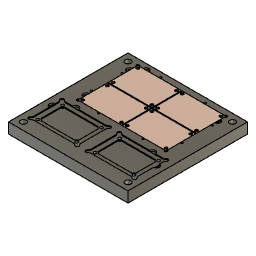
4x6 PCB jig (Autodesk Fusion 360 design; units mm, degrees)
Autodesk Fusion 360 part; units mm, degrees
sketch "Sketch1" plane through (0, 0, 0) normal (0, 0, 1) x (1, 0, 0) in component "holder"
  line L0 (0, 0) -> (203.2, 0)
  line L1 (203.2, 0) -> (203.2, 203.2)
  line L2 (203.2, 203.2) -> (0, 203.2)
  line L3 (0, 203.2) -> (0, 0)
  circle A0 centre (12.7, 12.7) radius 3
  circle A1 centre (190.5, 12.7) radius 3
  circle A2 centre (12.7, 190.5) radius 3
  circle A3 centre (190.5, 190.5) radius 3
  circle A4 centre (12.7, 12.7) radius 5
  circle A5 centre (190.5, 12.7) radius 5
  circle A6 centre (12.7, 190.5) radius 5
  circle A7 centre (190.5, 190.5) radius 5
  dimension "d1" = 203.2
  dimension "d2" = 203.2
  dimension "d3" = 6
  dimension "d4" = 12.7
  dimension "d5" = 12.7
  dimension "d8" = 177.8
  dimension "d9" = 177.8
  dimension "d12" = 10
  dimension "d15" = 177.8
  dimension "d16" = 177.8
  constraint horizontal L0
  constraint vertical L1
  constraint horizontal L2
  constraint vertical L3
  constraint coincident L0.start L3.end
  constraint concentric A0 A4
  measures "d1" distance of L0.start L0.end
  measures "d2" distance of L0.start L2.end
  measures "d3" diameter of A0
  measures "d4" distance of L3 A0.centre
  measures "d5" distance of L0 A0.centre
  measures "d12" diameter of A4
extrude "Extrude1" add sketch "Sketch1" along normal blind 17.9 contours L0 L1 L2 L3 | A4 | A5 | A6 | A7 makes body 1 in component "holder"
extrude "Extrude2" cut sketch "Sketch1" against normal blind 6.5 from surface at 17.9 contours A4 | A5 | A6 | A7 bodies 1 in component "holder"
sketch "Sketch2" plane through (0, 0, 17.9) normal (0, 0, 1) x (-1, 0, 0) in component "holder"
  circle A0 centre (-190.5, -12.7) radius 5
  circle A1 centre (-190.5, -190.5) radius 5
  circle A2 centre (-12.7, -12.7) radius 5
  circle A3 centre (-12.7, -190.5) radius 5
  line L0 (0, -203.2) -> (0, 0)
  line L1 (0, 0) -> (-203.2, 0)
  line L2 (-203.2, 0) -> (-203.2, -203.2)
  line L3 (-203.2, -203.2) -> (0, -203.2)
  line L4 (-26.7, -193.2) -> (-176.5, -193.2)
  line L5 (-176.5, -193.2) -> (-176.5, -91.3)
  line L6 (-176.5, -91.3) -> (-26.7, -91.3)
  line L7 (-26.7, -91.3) -> (-26.7, -193.2)
  line L8 (0, -203.2) -> (0, 0)
  line L9 (0, 0) -> (-203.2, 0)
  line L10 (-203.2, -203.2) -> (0, -203.2)
  line L11 (-13, -78) -> (-93, -78) construction
  line L12 (-93, -78) -> (-93, -24) construction
  line L13 (-93, -24) -> (-13, -24) construction
  line L14 (-13, -24) -> (-13, -78) construction
  line L15 (-101.6, -203.2) -> (-101.6, 0)
  line L16 (-53, -78) -> (-53, -24) construction
  line L17 (-13, -51) -> (-93, -51) construction
  line L18 (-13, -51) -> (-13.0014, -30.2465)
  line L19 (-53, -24) -> (-19.2578, -24.0135)
  arc A4 (-11.1255, -26.3423) -> (-15.3459, -22.1301) centre (-13, -24) ccw
  arc A5 (-11.1255, -26.3423) -> (-13.0014, -30.2465) centre (-8.0014, -30.2461) ccw
  arc A6 (-19.2578, -24.0135) -> (-15.3459, -22.1301) centre (-19.2558, -19.0135) ccw
  line L20 (-93, -51) -> (-92.9986, -30.2465)
  arc A7 (-92.9986, -30.2465) -> (-94.8745, -26.3423) centre (-97.9986, -30.2461) ccw
  arc A8 (-90.6541, -22.1301) -> (-94.8745, -26.3423) centre (-93, -24) ccw
  arc A9 (-90.6541, -22.1301) -> (-86.7422, -24.0135) centre (-86.7442, -19.0135) ccw
  line L21 (-53, -24) -> (-86.7422, -24.0135)
  line L22 (-53, -78) -> (-86.7422, -77.9865)
  arc A10 (-86.7422, -77.9865) -> (-90.6541, -79.8699) centre (-86.7442, -82.9865) ccw
  arc A11 (-94.8745, -75.6577) -> (-90.6541, -79.8699) centre (-93, -78) ccw
  arc A12 (-94.8745, -75.6577) -> (-92.9986, -71.7535) centre (-97.9986, -71.7539) ccw
  line L23 (-93, -51) -> (-92.9986, -71.7535)
  line L24 (-13, -51) -> (-13.0014, -71.7535)
  arc A13 (-13.0014, -71.7535) -> (-11.1255, -75.6577) centre (-8.0014, -71.7539) ccw
  arc A14 (-15.3459, -79.8699) -> (-19.2578, -77.9865) centre (-19.2558, -82.9865) ccw
  line L25 (-53, -78) -> (-19.2578, -77.9865)
  arc A15 (-15.3459, -79.8699) -> (-11.1255, -75.6577) centre (-13, -78) ccw
  line L26 (-26.7, -142.25) -> (-176.5, -142.25) construction
  arc A16 (-28.7, -193.2) -> (-26.7, -191.2) centre (-26.7, -193.2) ccw
  arc A17 (-176.5, -191.2) -> (-174.5, -193.2) centre (-176.5, -193.2) ccw
  arc A18 (-174.5, -91.3) -> (-176.5, -93.3) centre (-176.5, -91.3) ccw
  arc A19 (-26.7, -93.3) -> (-28.7, -91.3) centre (-26.7, -91.3) ccw
  circle A20 centre (-24.94, -168.1) radius 1.675
  line L27 (-26.7, -168.1) -> (-176.5, -168.1) construction
  line L28 (-63.775, -193.2) -> (-63.775, -91.3) construction
  line L29 (-26.7, -168.1) -> (-16.7, -168.1) construction
  line L30 (-63.775, -193.2) -> (-63.775, -203.2) construction
  circle A21 centre (-63.775, -194.96) radius 1.675
  circle A22 centre (-63.775, -89.54) radius 1.675
  circle A23 centre (-24.94, -116.4) radius 1.675
  circle A24 centre (-139.425, -194.96) radius 1.675
  circle A25 centre (-178.26, -168.1) radius 1.675
  circle A26 centre (-178.26, -116.4) radius 1.675
  circle A27 centre (-139.425, -89.54) radius 1.675
  circle A28 centre (-30.775, -189.1) radius 2.425
  circle A29 centre (-96.775, -189.1) radius 2.425
  circle A30 centre (-30.775, -147.1) radius 2.425
  circle A31 centre (-96.775, -147.1) radius 2.425
  line L31 (-100.85, -193.2) -> (-100.85, -91.3) construction
  arc A32 (-100.85, -91.3) -> (-102.35, -91.3) centre (-101.6, -91.3) ccw construction
  line L32 (-102.35, -91.3) -> (-102.35, -193.2) construction
  arc A33 (-102.35, -193.2) -> (-100.85, -193.2) centre (-101.6, -193.2) ccw construction
  line L33 (-101.6, -193.2) -> (-101.6, -91.3) construction
  line L34 (-26.7, -141.5) -> (-176.5, -141.5) construction
  arc A34 (-176.5, -141.5) -> (-176.5, -143) centre (-176.5, -142.25) ccw construction
  line L35 (-176.5, -143) -> (-26.7, -143) construction
  arc A35 (-26.7, -143) -> (-26.7, -141.5) centre (-26.7, -142.25) ccw construction
  line L36 (-26.7, -142.25) -> (-176.5, -142.25)
  circle A36 centre (-172.425, -189.1) radius 2.425
  circle A37 centre (-106.425, -189.1) radius 2.425
  circle A38 centre (-106.425, -147.1) radius 2.425
  circle A39 centre (-172.425, -147.1) radius 2.425
  circle A40 centre (-30.775, -95.4) radius 2.425
  circle A41 centre (-96.775, -95.4) radius 2.425
  circle A42 centre (-106.425, -95.4) radius 2.425
  circle A43 centre (-172.425, -95.4) radius 2.425
  circle A44 centre (-172.425, -137.4) radius 2.425
  circle A45 centre (-106.425, -137.4) radius 2.425
  circle A46 centre (-96.775, -137.4) radius 2.425
  circle A47 centre (-30.775, -137.4) radius 2.425
  circle A48 centre (-20, -72) radius 2.425
  circle A49 centre (-86, -72) radius 2.425
  circle A50 centre (-20, -30) radius 2.425
  circle A51 centre (-86, -30) radius 2.425
  line L37 (-150.2, -78) -> (-183.9422, -77.9865)
  arc A52 (-183.9422, -77.9865) -> (-187.8541, -79.8699) centre (-183.9442, -82.9865) ccw
  arc A53 (-192.0745, -75.6577) -> (-190.1986, -71.7535) centre (-195.1986, -71.7539) ccw
  line L38 (-190.2, -51) -> (-190.1986, -71.7535)
  arc A54 (-192.0745, -75.6577) -> (-187.8541, -79.8699) centre (-190.2, -78) ccw
  line L39 (-110.2, -51) -> (-110.2014, -71.7535)
  arc A55 (-110.2014, -71.7535) -> (-108.3255, -75.6577) centre (-105.2014, -71.7539) ccw
  arc A56 (-112.5459, -79.8699) -> (-116.4578, -77.9865) centre (-116.4558, -82.9865) ccw
  line L40 (-150.2, -78) -> (-116.4578, -77.9865)
  arc A57 (-112.5459, -79.8699) -> (-108.3255, -75.6577) centre (-110.2, -78) ccw
  line L41 (-150.2, -24) -> (-116.4578, -24.0135)
  arc A58 (-116.4578, -24.0135) -> (-112.5459, -22.1301) centre (-116.4558, -19.0135) ccw
  arc A59 (-108.3255, -26.3423) -> (-110.2014, -30.2465) centre (-105.2014, -30.2461) ccw
  line L42 (-110.2, -51) -> (-110.2014, -30.2465)
  arc A60 (-108.3255, -26.3423) -> (-112.5459, -22.1301) centre (-110.2, -24) ccw
  line L43 (-190.2, -51) -> (-190.1986, -30.2465)
  arc A61 (-190.1986, -30.2465) -> (-192.0745, -26.3423) centre (-195.1986, -30.2461) ccw
  arc A62 (-187.8541, -22.1301) -> (-183.9422, -24.0135) centre (-183.9442, -19.0135) ccw
  line L44 (-150.2, -24) -> (-183.9422, -24.0135)
  arc A63 (-187.8541, -22.1301) -> (-192.0745, -26.3423) centre (-190.2, -24) ccw
  circle A64 centre (-183.2, -30) radius 2.425
  circle A65 centre (-183.2, -72) radius 2.425
  circle A66 centre (-117.2, -72) radius 2.425
  circle A67 centre (-117.2, -30) radius 2.425
  circle A68 centre (-20, -72) radius 3.545
  circle A69 centre (-86, -72) radius 3.545
  circle A70 centre (-20, -30) radius 3.545
  circle A71 centre (-86, -30) radius 3.545
  circle A72 centre (-183.2, -72) radius 3.545
  circle A73 centre (-117.2, -72) radius 3.545
  circle A74 centre (-117.2, -30) radius 3.545
  circle A75 centre (-183.2, -30) radius 3.545
  line L45 (-27.6816, -194.9425) -> (-30.775, -193.2)
  line L46 (-24.9541, -192.2244) -> (-26.7, -189.1)
  line L47 (-175.5184, -194.9425) -> (-172.425, -193.2)
  line L48 (-178.2459, -192.2244) -> (-176.5, -189.1)
  line L49 (-24.9541, -92.2756) -> (-26.7, -95.4)
  line L50 (-27.6816, -89.5575) -> (-30.775, -91.3)
  line L51 (-175.5184, -89.5575) -> (-172.425, -91.3)
  line L52 (-178.2459, -92.2756) -> (-176.5, -95.4)
  dimension "d20" = 149.8
  dimension "d21" = 101.9
  dimension "d24" = 10
  dimension "d25" = 80
  dimension "d26" = 54
  dimension "d30" = 6
  dimension "d31" = 5
  dimension "d32" = 4
  dimension "d33" = 3.35
  dimension "d34" = 1.76
  dimension "d37" = 1.76
  dimension "d38" = 4.85
  dimension "d39" = 66
  dimension "d40" = 42
  dimension "d41" = 1.5
  dimension "d42" = 1.5
  dimension "d43" = 66
  dimension "d44" = 42
  dimension "d45" = 20
  dimension "d46" = 30
  dimension "d47" = 7.09
  constraint horizontal L4
  constraint vertical L5
  constraint horizontal L6
  constraint vertical L7
  constraint horizontal L11
  constraint vertical L12
  constraint horizontal L13
  constraint vertical L14
  constraint midpoint L3 L15.start
  constraint midpoint L1 L15.end
  constraint midpoint L11 L16.start
  constraint midpoint L13 L16.end
  constraint midpoint L14 L17.start
  constraint midpoint L12 L17.end
  constraint coincident L13.end L14.start
  constraint tangent L18 A5
  constraint tangent A4 A5
  constraint tangent L19 A6
  constraint tangent A4 A6
  constraint equal A5 A6
  constraint symmetric L19.start L16 L21.start
  constraint symmetric L16 L17.start L17.end
  constraint symmetric L16 A4 A8
  constraint symmetric L16 L18.end L20.end
  constraint symmetric L16 A4.start A7.end
  constraint symmetric L16 A5 A7
  constraint symmetric L16 L19.end A9.end
  constraint symmetric L16 A4.end A8.start
  constraint symmetric L16 A6 A9
  constraint symmetric L16.end L17 L16.start
  constraint symmetric L18.start L17 L24.start
  constraint symmetric L17 A4 A15
  constraint symmetric L17 L18.end L24.end
  constraint symmetric L17 A4.start A13.end
  constraint symmetric L17 A5 A13
  constraint symmetric L17 L19.end A14.end
  constraint symmetric L17 A4.end A14.start
  constraint symmetric L17 A6 A14
  constraint symmetric L17 L20.start L23.start
  constraint symmetric L17 L20.end A12.end
  constraint symmetric L17 A7.end A11.start
  constraint symmetric L17 A7 A12
  constraint symmetric L17 A8.start A10.end
  constraint symmetric L17 A8 A11
  constraint symmetric L17 A9.end L22.end
  constraint symmetric L17 A9 A10
  constraint symmetric L17 L16.end L16.start
  constraint symmetric L5 L7 L15
  constraint coincident L4.start L7.end
  constraint symmetric L15 A16 A17
  constraint midpoint L7 L26.start
  constraint midpoint L5 L26.end
  constraint symmetric L26 A16 A19
  constraint symmetric L26 A17 A18
  constraint coincident L7 A16.end
  constraint coincident L4 A16.start
  constraint coincident L4 A17.end
  constraint coincident L5 A17.start
  constraint coincident L5 A18.end
  constraint coincident L6 A18.start
  constraint coincident L6 A19.end
  constraint coincident L7 A19.start
  constraint coincident L7 L27.start
  constraint coincident L5 L27.end
  constraint perpendicular L5 L27
  constraint coincident L4 L28.start
  constraint coincident L6 L28.end
  constraint perpendicular L7 L29
  constraint perpendicular L4 L30
  constraint coincident A20.centre L29
  constraint equal A20 A21
  constraint coincident L30 A21.centre
  constraint symmetric L26 A20 A23
  constraint symmetric L26 A21 A22
  constraint symmetric L15 A20 A25
  constraint symmetric L15 A21 A24
  constraint symmetric L15 A22 A27
  constraint symmetric L15 A23 A26
  constraint symmetric L27 A28 A30
  constraint tangent L31 A32
  constraint tangent A32 L32
  constraint parallel L31 L32
  constraint tangent L32 A33
  constraint tangent L31 A33
  constraint midpoint L6 A32.centre
  constraint perpendicular L6 L33
  constraint midpoint L4 A33.centre
  constraint tangent L34 A34
  constraint tangent A34 L35
  constraint parallel L34 L35
  constraint tangent L35 A35
  constraint tangent L34 A35
  constraint coincident L26.end A34.centre
  constraint perpendicular L5 L36
  constraint coincident L26.start A35.centre
  constraint symmetric L4 L27 L35
  constraint symmetric L28 A28.centre A29.centre
  constraint equal A28 A29
  constraint equal A28 A31
  constraint vertical A29.centre A31.centre
  constraint horizontal A30.centre A31.centre
  constraint symmetric L15 A28 A36
  constraint symmetric L15 A29 A37
  constraint symmetric L15 A30 A39
  constraint symmetric L15 A31 A38
  constraint symmetric A28 L36 A40
  constraint symmetric A29 L36 A41
  constraint symmetric A30 L36 A47
  constraint symmetric A31 L36 A46
  constraint symmetric L36 A36 A43
  constraint symmetric L36 A37 A42
  constraint symmetric L36 A38 A45
  constraint symmetric L36 A39 A44
  constraint equal A28 A48
  constraint symmetric L16 A48 A49
  constraint symmetric L17 A48 A50
  constraint symmetric L17 A49 A51
  constraint symmetric L15 L16.end L41.start
  constraint symmetric L15 L17.start L38.start
  constraint symmetric L15 A4 A63
  constraint symmetric L15 L18.end L43.end
  constraint symmetric L15 A4.start A61.end
  constraint symmetric L15 A5 A61
  constraint symmetric L15 L19.end A62.end
  constraint symmetric L15 A4.end A62.start
  constraint symmetric L15 A6 A62
  constraint symmetric L15 L17.end L39.start
  constraint symmetric L15 L20.end A59.end
  constraint symmetric L15 A7.end A59.start
  constraint symmetric L15 A7 A59
  constraint symmetric L15 A8.start A58.end
  constraint symmetric L15 A8 A60
  constraint symmetric L15 A9.end L41.end
  constraint symmetric L15 A9 A58
  constraint symmetric L15 L16.start L37.start
  constraint symmetric L15 L22.end A56.end
  constraint symmetric L15 A10.end A56.start
  constraint symmetric L15 A10 A56
  constraint symmetric L15 A11.start A55.end
  constraint symmetric L15 A11 A57
  constraint symmetric L15 A12.end L39.end
  constraint symmetric L15 A12 A55
  constraint symmetric L15 L24.end A53.end
  constraint symmetric L15 A13.end A53.start
  constraint symmetric L15 A13 A53
  constraint symmetric L15 A14.end L37.end
  constraint symmetric L15 A14.start A52.end
  constraint symmetric L15 A14 A52
  constraint symmetric L15 A15 A54
  constraint symmetric L15 A48 A65
  constraint symmetric L15 A49 A66
  constraint symmetric L15 A50 A64
  constraint symmetric L15 A51 A67
  constraint concentric A48 A68
  constraint symmetric L16 A68 A69
  constraint symmetric L17 A68 A70
  constraint symmetric L17 A69 A71
  constraint symmetric L15 A68 A72
  constraint symmetric L15 A69 A73
  constraint symmetric L15 A70 A75
  constraint symmetric L15 A71 A74
  constraint coincident A16 L45.start
  constraint coincident L4 L45.end
  constraint tangent A16 L45
  constraint vertical A28.centre L45.end
  constraint coincident A16 L46.start
  constraint tangent A16 L46
  constraint horizontal A28.centre L46.end
  constraint coincident L7 L46.end
  constraint symmetric L15 L45.start L47.start
  constraint symmetric L15 L45.end L47.end
  constraint symmetric L15 L46.start L48.start
  constraint symmetric L15 L46.end L48.end
  constraint symmetric L26 L45.start L50.start
  constraint symmetric L26 L45.end L50.end
  constraint symmetric L26 L46.start L49.start
  constraint symmetric L26 L46.end L49.end
  constraint symmetric L26 L47.start L51.start
  constraint symmetric L26 L47.end L51.end
  constraint symmetric L26 L48.start L52.start
  constraint symmetric L26 L48.end L52.end
  measures "d20" distance of L4.start L4.end
  measures "d21" distance of L4.start L6.end
  measures "d24" distance of L4 L10
  measures "d25" distance of L11.start L11.end
  measures "d26" distance of L11.start L13.end
  measures "d30" diameter of A4
  measures "d31" radius of A5
  measures "d32" diameter of A16
  measures "d33" diameter of A20
  measures "d34" distance of L7 A20.centre
  measures "d37" vertical distance of L28.start A21.centre
  measures "d38" diameter of A28
  measures "d39" distance of A28.centre A29.centre
  measures "d40" distance of A28.centre A30.centre
  measures "d41" diameter of A32
  measures "d42" diameter of A34
  measures "d43" distance of A48.centre A49.centre
  measures "d44" distance of A48.centre A50.centre
  measures "d45" distance of L8 A50.centre
  measures "d46" distance of L9 A50.centre
  measures "d47" diameter of A68
extrude "Extrude3" cut sketch "Sketch2" against normal blind 1.5 contours L4 L7 L15 L36 | L4 L5 L15 L36 | L5 L6 L15 L36 | L6 L7 L15 L36 | L4 A16 L45 | L4 A17 L47 | L6 A18 L51 | L6 A19 L50 | L4 L7 A16 | L4 L5 A17 | L5 L6 A18 | L6 L7 A19 | L7 A16 L46 | L5 A17 L48 | L7 A19 L49 | L5 A18 L52 | L18 L19 A4 A5 A6 L20 A7 A8 A9 L21 L22 A10 A11 A12 L23 L24 A13 A14 L25 A15 | A28 | A29 | A30 | A31 | A36 | A37 | A38 | A39 | A40 | A41 | A42 | A43 | A44 | A45 | A46 | A47 | A48 | A49 | A50 | A51 | L37 A52 A53 L38 A54 L39 A55 A56 L40 A57 L41 A58 A59 L42 A60 L43 A61 A62 L44 A63 | A64 | A65 | A66 | A67 | A68 | A69 | A70 | A71 | A72 | A73 | A74 | A75 bodies 1 in component "holder"
sketch "Sketch1 (2)" plane through (0, 0, 0) normal (1, 0, 0) x (0, 1, 0)
extrude "Extrude4" cut sketch "Sketch2" against normal blind 12 contours A20 | A21 | A22 | A23 | A24 | A25 | A26 | A27 bodies 1 in component "holder"
extrude "Extrude5" cut sketch "Sketch2" against normal blind 4 contours A28 | A29 | A30 | A31 | A36 | A37 | A38 | A39 | A40 | A41 | A42 | A43 | A44 | A45 | A46 | A47 bodies 1 in component "holder"
extrude "Extrude6" cut sketch "Sketch2" against normal up to surface (17.9 mm away) contours A48 | A49 | A50 | A51 | A64 | A65 | A66 | A67 bodies 1 in component "holder"
extrude "Extrude7" cut sketch "Sketch2" along normal blind 9.5 from surface at -17.9 contours A68 | A69 | A70 | A71 | A72 | A73 | A74 | A75 bodies 1 in component "holder"
sketch "Sketch2 (2)" plane through (0, 0, 0) normal (0, 0, -1) x (1, 0, 0)
  circle A0 centre (117.2, -30) radius 3.545
  circle A1 centre (86, -72) radius 3.545
  circle A2 centre (86, -30) radius 3.545
  circle A3 centre (183.2, -30) radius 3.545
  circle A4 centre (117.2, -72) radius 3.545
  circle A5 centre (20, -72) radius 3.545
  circle A6 centre (20, -30) radius 3.545
  circle A7 centre (183.2, -72) radius 3.545
  circle A8 centre (12.7, -190.5) radius 3
  circle A9 centre (190.5, -190.5) radius 3
  circle A10 centre (190.5, -12.7) radius 3
  circle A11 centre (12.7, -12.7) radius 3
  line L0 (0, 0) -> (0, -203.2)
  line L1 (0, -203.2) -> (203.2, -203.2)
  line L2 (203.2, -203.2) -> (203.2, 0)
  line L3 (203.2, 0) -> (0, 0)
sketch "Sketch3" plane through (0, 0, 17.9) normal (0, 0, 1) x (-1, 0, 0)
  line L0 (-26.7, -91.3) -> (-26.7, -193.2)
  line L1 (-13, -51) -> (-13.0014, -71.7535)
  line L2 (-53, -78) -> (-19.2578, -77.9865)
  line L3 (-190.2, -51) -> (-190.1986, -71.7535)
  line L4 (-150.2, -78) -> (-183.9422, -77.9865)
  line L5 (-176.5, -91.3) -> (-26.7, -91.3)
  line L6 (-176.5, -193.2) -> (-176.5, -91.3)
  line L7 (-53, -24) -> (-19.2578, -24.0135)
  line L8 (-13, -24) -> (-13, -78)
  line L9 (-150.2, -24) -> (-183.9422, -24.0135)
  line L10 (-190.2, -51) -> (-190.1986, -30.2465)
  circle A0 centre (-26.7, -179.2) radius 5
  line L11 (-26.7, -193.2) -> (-176.5, -193.2)
  circle A1 centre (-40.7, -193.2) radius 5
  circle A2 centre (-26.7, -105.3) radius 5
  circle A3 centre (-13.0007, -61.3768) radius 5
  circle A4 centre (-36.1289, -77.9932) radius 5
  circle A5 centre (-167.0711, -77.9932) radius 5
  circle A6 centre (-190.1993, -61.3768) radius 5
  circle A7 centre (-176.5, -179.2) radius 5
  dimension "d59" = 10
  dimension "d60" = 14
  dimension "d61" = 10
  dimension "d62" = 14
  dimension "d63" = 10
  dimension "d64" = 14
  dimension "d65" = 10
  dimension "d66" = 10
  dimension "d67" = 10
  dimension "d68" = 10
  dimension "d69" = 10
  constraint coincident L0 A0.centre
  constraint coincident L11 A1.centre
  constraint coincident L0 A2.centre
  constraint midpoint L1 A3.centre
  constraint midpoint L2 A4.centre
  constraint midpoint L4 A5.centre
  constraint midpoint L3 A6.centre
  constraint coincident L6 A7.centre
  constraint horizontal A0.centre A7.centre
  measures "d59" diameter of A0
  measures "d60" distance of A0.centre L11
  measures "d61" diameter of A1
  measures "d62" distance of L0 A1.centre
  measures "d63" diameter of A2
  measures "d64" distance of L5 A2.centre
  measures "d65" diameter of A3
  measures "d66" diameter of A4
  measures "d67" diameter of A5
  measures "d68" diameter of A6
  measures "d69" diameter of A7
extrude "Extrude8" cut sketch "Sketch3" against normal blind 2.5 contours L0 A2 | L6 A7 | L0 A0 | L11 A1 | L8 A3 | L2 A4 | L3 A6 | L4 A5 picked at (-24.7337, -106.442) picked at (-177.4715, -180.683) picked at (-23.6872, -180.4506) picked at (-42.1373, -195.7637) picked at (-34.8883, -79.3751) picked at (-191.3865, -62.7725) picked at (-165.7533, -81.1536) bodies 1 in component "holder"
sketch "Sketch3 (2)" plane through (0, 0, 16.4) normal (0, 0, 1) x (-1, 0, 0) in component "holder"
  circle A0 centre (-30.775, -95.4) radius 2.425
  circle A1 centre (-106.425, -189.1) radius 2.425
  circle A2 centre (-172.425, -189.1) radius 2.425
  circle A3 centre (-96.775, -189.1) radius 2.425
  circle A4 centre (-30.775, -147.1) radius 2.425
  circle A5 centre (-172.425, -137.4) radius 2.425
  circle A6 centre (-96.775, -147.1) radius 2.425
  circle A7 centre (-96.775, -95.4) radius 2.425
  circle A8 centre (-172.425, -95.4) radius 2.425
  circle A9 centre (-30.775, -189.1) radius 2.425
  circle A10 centre (-106.425, -147.1) radius 2.425
  circle A11 centre (-30.775, -137.4) radius 2.425
  circle A12 centre (-172.425, -147.1) radius 2.425
  circle A13 centre (-106.425, -137.4) radius 2.425
  circle A14 centre (-96.775, -137.4) radius 2.425
  circle A15 centre (-106.425, -95.4) radius 2.425
  arc A16 (-175.5184, -89.5575) -> (-178.2459, -92.2756) centre (-176.5, -91.3) ccw
  line L0 (-178.2459, -92.2756) -> (-176.5, -95.4)
  line L1 (-176.5, -95.4) -> (-176.5, -174.2)
  line L2 (-176.5, -174.2) -> (-176.5, -184.2)
  line L3 (-176.5, -184.2) -> (-176.5, -189.1)
  line L4 (-176.5, -189.1) -> (-178.2459, -192.2244)
  arc A17 (-178.2459, -192.2244) -> (-175.5184, -194.9425) centre (-176.5, -193.2) ccw
  line L5 (-175.5184, -194.9425) -> (-172.425, -193.2)
  line L6 (-172.425, -193.2) -> (-45.7, -193.2)
  line L7 (-45.7, -193.2) -> (-35.7, -193.2)
  line L8 (-35.7, -193.2) -> (-30.775, -193.2)
  line L9 (-30.775, -193.2) -> (-27.6816, -194.9425)
  arc A18 (-27.6816, -194.9425) -> (-24.9541, -192.2244) centre (-26.7, -193.2) ccw
  line L10 (-24.9541, -192.2244) -> (-26.7, -189.1)
  line L11 (-26.7, -189.1) -> (-26.7, -184.2)
  line L12 (-26.7, -184.2) -> (-26.7, -174.2)
  line L13 (-26.7, -174.2) -> (-26.7, -110.3)
  line L14 (-26.7, -110.3) -> (-26.7, -100.3)
  line L15 (-26.7, -100.3) -> (-26.7, -95.4)
  line L16 (-26.7, -95.4) -> (-24.9541, -92.2756)
  arc A19 (-24.9541, -92.2756) -> (-27.6816, -89.5575) centre (-26.7, -91.3) ccw
  line L17 (-27.6816, -89.5575) -> (-30.775, -91.3)
  line L18 (-30.775, -91.3) -> (-172.425, -91.3)
  line L19 (-172.425, -91.3) -> (-175.5184, -89.5575)
  line L20 (-26.7, -91.3) -> (-26.7, -193.2)
  line L21 (-26.7, -193.2) -> (-176.5, -193.2)
  line L22 (-176.5, -193.2) -> (-176.5, -91.3)
  line L23 (-176.5, -91.3) -> (-26.7, -91.3)
  line L24 (-26.7, -142.25) -> (-176.5, -142.25)
  line L25 (-101.6, -193.2) -> (-101.6, -91.3)
  circle A20 centre (-30.775, -189.1) radius 2.425
  circle A21 centre (-96.775, -189.1) radius 2.425
  circle A22 centre (-106.425, -189.1) radius 2.425
  circle A23 centre (-172.425, -189.1) radius 2.425
  circle A24 centre (-172.425, -147.1) radius 2.425
  circle A25 centre (-172.425, -137.4) radius 2.425
  circle A26 centre (-172.425, -95.4) radius 2.425
  circle A27 centre (-106.425, -95.4) radius 2.425
  circle A28 centre (-106.425, -137.4) radius 2.425
  circle A29 centre (-106.425, -147.1) radius 2.425
  circle A30 centre (-96.775, -147.1) radius 2.425
  circle A31 centre (-96.775, -137.4) radius 2.425
  circle A32 centre (-96.775, -95.4) radius 2.425
  circle A33 centre (-30.775, -95.4) radius 2.425
  circle A34 centre (-30.775, -137.4) radius 2.425
  circle A35 centre (-30.775, -147.1) radius 2.425
  line L26 (-176.5, -143) -> (-26.7, -143)
  line L27 (-26.7, -141.5) -> (-176.5, -141.5)
  line L28 (-100.85, -193.2) -> (-100.85, -91.3)
  line L29 (-102.35, -91.3) -> (-102.35, -193.2)
  line L30 (-27.1412, -143) -> (-27.1412, -141.5)
  line L31 (-100.85, -192.6157) -> (-102.35, -192.6157)
  line L32 (-175.8243, -143) -> (-175.8243, -141.5)
  line L33 (-100.85, -92.2176) -> (-102.35, -92.2176)
  constraint coincident L26 L30.start
  constraint coincident L27 L30.end
  constraint perpendicular L27 L30
  constraint coincident L28 L31.start
  constraint coincident L29 L31.end
  constraint perpendicular L29 L31
  constraint coincident L26 L32.start
  constraint coincident L27 L32.end
  constraint perpendicular L27 L32
  constraint coincident L28 L33.start
  constraint coincident L29 L33.end
  constraint perpendicular L29 L33
extrude "Extrude9" add sketch "Sketch3 (2)" along normal blind 1.5 separate body contours L1 L18 L22 L23 L27 L29 | L18 L23 L25 L29 L33 | L1 L22 L24 L27 L32 | L18 L23 L25 L28 L33 | L1 L22 L24 L26 L32 | L13 L14 L15 L18 L20 L23 L27 L28 | L1 L2 L3 L6 L21 L22 L26 L29 | L13 L20 L24 L27 L30 | L6 L21 L25 L29 L31 | L13 L20 L24 L26 L30 | L6 L7 L8 L11 L12 L13 L20 L21 L26 L28 | L6 L21 L25 L28 L31 makes body 2 in component "holder"
sketch "Sketch4" plane through (0, 0, 17.9) normal (0, 0, 1) x (-1, 0, 0) in component "holder"
  line L0 (0, -203.2) -> (0, 0)
  line L1 (0, 0) -> (-203.2, 0)
  line L2 (-203.2, 0) -> (-203.2, -203.2)
  line L3 (-203.2, -203.2) -> (0, -203.2)
  circle A0 centre (-12.7, -190.5) radius 5
  circle A1 centre (-12.7, -12.7) radius 5
  circle A2 centre (-190.5, -190.5) radius 5
  circle A3 centre (-190.5, -12.7) radius 5
  arc A4 (-172.0711, -77.9912) -> (-162.0711, -77.9952) centre (-167.0711, -77.9932) ccw
  line L4 (-172.0711, -77.9912) -> (-183.9422, -77.9865)
  arc A5 (-183.9422, -77.9865) -> (-187.8541, -79.8699) centre (-183.9442, -82.9865) ccw
  arc A6 (-192.0745, -75.6577) -> (-187.8541, -79.8699) centre (-190.2, -78) ccw
  arc A7 (-192.0745, -75.6577) -> (-190.1986, -71.7535) centre (-195.1986, -71.7539) ccw
  line L5 (-190.1986, -71.7535) -> (-190.199, -66.3768)
  arc A8 (-190.1996, -56.3768) -> (-190.199, -66.3768) centre (-190.1993, -61.3768) ccw
  line L6 (-190.1996, -56.3768) -> (-190.2, -51)
  line L7 (-190.2, -51) -> (-190.1986, -30.2465)
  arc A9 (-190.1986, -30.2465) -> (-192.0745, -26.3423) centre (-195.1986, -30.2461) ccw
  arc A10 (-187.8541, -22.1301) -> (-192.0745, -26.3423) centre (-190.2, -24) ccw
  arc A11 (-187.8541, -22.1301) -> (-183.9422, -24.0135) centre (-183.9442, -19.0135) ccw
  line L8 (-183.9422, -24.0135) -> (-150.2, -24)
  line L9 (-150.2, -24) -> (-116.4578, -24.0135)
  arc A12 (-116.4578, -24.0135) -> (-112.5459, -22.1301) centre (-116.4558, -19.0135) ccw
  arc A13 (-108.3255, -26.3423) -> (-112.5459, -22.1301) centre (-110.2, -24) ccw
  arc A14 (-108.3255, -26.3423) -> (-110.2014, -30.2465) centre (-105.2014, -30.2461) ccw
  line L10 (-110.2014, -30.2465) -> (-110.2, -51)
  line L11 (-110.2, -51) -> (-110.2014, -71.7535)
  arc A15 (-110.2014, -71.7535) -> (-108.3255, -75.6577) centre (-105.2014, -71.7539) ccw
  arc A16 (-112.5459, -79.8699) -> (-108.3255, -75.6577) centre (-110.2, -78) ccw
  arc A17 (-112.5459, -79.8699) -> (-116.4578, -77.9865) centre (-116.4558, -82.9865) ccw
  line L12 (-116.4578, -77.9865) -> (-150.2, -78)
  line L13 (-150.2, -78) -> (-162.0711, -77.9952)
  arc A18 (-41.1289, -77.9952) -> (-31.1289, -77.9912) centre (-36.1289, -77.9932) ccw
  line L14 (-41.1289, -77.9952) -> (-53, -78)
  line L15 (-53, -78) -> (-86.7422, -77.9865)
  arc A19 (-86.7422, -77.9865) -> (-90.6541, -79.8699) centre (-86.7442, -82.9865) ccw
  arc A20 (-94.8745, -75.6577) -> (-90.6541, -79.8699) centre (-93, -78) ccw
  arc A21 (-94.8745, -75.6577) -> (-92.9986, -71.7535) centre (-97.9986, -71.7539) ccw
  line L16 (-92.9986, -71.7535) -> (-93, -51)
  line L17 (-93, -51) -> (-92.9986, -30.2465)
  arc A22 (-92.9986, -30.2465) -> (-94.8745, -26.3423) centre (-97.9986, -30.2461) ccw
  arc A23 (-90.6541, -22.1301) -> (-94.8745, -26.3423) centre (-93, -24) ccw
  arc A24 (-90.6541, -22.1301) -> (-86.7422, -24.0135) centre (-86.7442, -19.0135) ccw
  line L18 (-86.7422, -24.0135) -> (-53, -24)
  line L19 (-53, -24) -> (-19.2578, -24.0135)
  arc A25 (-19.2578, -24.0135) -> (-15.3459, -22.1301) centre (-19.2558, -19.0135) ccw
  arc A26 (-11.1255, -26.3423) -> (-15.3459, -22.1301) centre (-13, -24) ccw
  arc A27 (-11.1255, -26.3423) -> (-13.0014, -30.2465) centre (-8.0014, -30.2461) ccw
  line L20 (-13.0014, -30.2465) -> (-13, -51)
  line L21 (-13, -51) -> (-13.0014, -71.7535)
  arc A28 (-13.0014, -71.7535) -> (-11.1255, -75.6577) centre (-8.0014, -71.7539) ccw
  arc A29 (-15.3459, -79.8699) -> (-11.1255, -75.6577) centre (-13, -78) ccw
  arc A30 (-15.3459, -79.8699) -> (-19.2578, -77.9865) centre (-19.2558, -82.9865) ccw
  line L22 (-19.2578, -77.9865) -> (-31.1289, -77.9912)
  arc A31 (-26.7, -184.2) -> (-26.7, -174.2) centre (-26.7, -179.2) ccw
  line L23 (-26.7, -184.2) -> (-26.7, -189.1)
  line L24 (-26.7, -189.1) -> (-24.9541, -192.2244)
  arc A32 (-27.6816, -194.9425) -> (-24.9541, -192.2244) centre (-26.7, -193.2) ccw
  line L25 (-27.6816, -194.9425) -> (-30.775, -193.2)
  line L26 (-30.775, -193.2) -> (-35.7, -193.2)
  arc A33 (-45.7, -193.2) -> (-35.7, -193.2) centre (-40.7, -193.2) ccw
  line L27 (-45.7, -193.2) -> (-172.425, -193.2)
  line L28 (-172.425, -193.2) -> (-175.5184, -194.9425)
  arc A34 (-178.2459, -192.2244) -> (-175.5184, -194.9425) centre (-176.5, -193.2) ccw
  line L29 (-178.2459, -192.2244) -> (-176.5, -189.1)
  line L30 (-176.5, -189.1) -> (-176.5, -184.2)
  arc A35 (-176.5, -174.2) -> (-176.5, -184.2) centre (-176.5, -179.2) ccw
  line L31 (-176.5, -174.2) -> (-176.5, -95.4)
  line L32 (-176.5, -95.4) -> (-178.2459, -92.2756)
  arc A36 (-175.5184, -89.5575) -> (-178.2459, -92.2756) centre (-176.5, -91.3) ccw
  line L33 (-175.5184, -89.5575) -> (-172.425, -91.3)
  line L34 (-172.425, -91.3) -> (-30.775, -91.3)
  line L35 (-30.775, -91.3) -> (-27.6816, -89.5575)
  arc A37 (-24.9541, -92.2756) -> (-27.6816, -89.5575) centre (-26.7, -91.3) ccw
  line L36 (-24.9541, -92.2756) -> (-26.7, -95.4)
  line L37 (-26.7, -95.4) -> (-26.7, -100.3)
  arc A38 (-26.7, -110.3) -> (-26.7, -100.3) centre (-26.7, -105.3) ccw
  line L38 (-26.7, -110.3) -> (-26.7, -174.2)
  circle A39 centre (-178.26, -168.1) radius 1.675
  circle A40 centre (-24.94, -116.4) radius 1.675
  circle A41 centre (-63.775, -194.96) radius 1.675
  circle A42 centre (-63.775, -89.54) radius 1.675
  circle A43 centre (-178.26, -116.4) radius 1.675
  circle A44 centre (-24.94, -168.1) radius 1.675
  circle A45 centre (-139.425, -194.96) radius 1.675
  circle A46 centre (-139.425, -89.54) radius 1.675
  line L39 (-13, -66.3768) -> (-13, -56.3768)
  arc A47 (-13, -66.3768) -> (-13, -56.3768) centre (-13.0007, -61.3768) ccw
  circle A48 centre (-86, -72) radius 2.425
  circle A49 centre (-86, -30) radius 2.425
  circle A50 centre (-20, -72) radius 2.425
  circle A51 centre (-20, -30) radius 2.425
  line L40 (-31.1289, -77.9912) -> (-19.2578, -77.9865)
  arc A52 (-15.3459, -79.8699) -> (-19.2578, -77.9865) centre (-19.2558, -82.9865) ccw
  arc A53 (-15.3459, -79.8699) -> (-11.1255, -75.6577) centre (-13, -78) ccw
  arc A54 (-13.0014, -71.7535) -> (-11.1255, -75.6577) centre (-8.0014, -71.7539) ccw
  line L41 (-13.0014, -71.7535) -> (-13, -51)
  line L42 (-13, -51) -> (-13.0014, -30.2465)
  arc A55 (-11.1255, -26.3423) -> (-13.0014, -30.2465) centre (-8.0014, -30.2461) ccw
  arc A56 (-11.1255, -26.3423) -> (-15.3459, -22.1301) centre (-13, -24) ccw
  arc A57 (-19.2578, -24.0135) -> (-15.3459, -22.1301) centre (-19.2558, -19.0135) ccw
  line L43 (-19.2578, -24.0135) -> (-53, -24)
  line L44 (-53, -24) -> (-86.7422, -24.0135)
  arc A58 (-90.6541, -22.1301) -> (-86.7422, -24.0135) centre (-86.7442, -19.0135) ccw
  arc A59 (-90.6541, -22.1301) -> (-94.8745, -26.3423) centre (-93, -24) ccw
  arc A60 (-92.9986, -30.2465) -> (-94.8745, -26.3423) centre (-97.9986, -30.2461) ccw
  line L45 (-92.9986, -30.2465) -> (-93, -51)
  line L46 (-93, -51) -> (-92.9986, -71.7535)
  arc A61 (-94.8745, -75.6577) -> (-92.9986, -71.7535) centre (-97.9986, -71.7539) ccw
  arc A62 (-94.8745, -75.6577) -> (-90.6541, -79.8699) centre (-93, -78) ccw
  arc A63 (-86.7422, -77.9865) -> (-90.6541, -79.8699) centre (-86.7442, -82.9865) ccw
  line L47 (-86.7422, -77.9865) -> (-53, -78)
  line L48 (-53, -78) -> (-41.1289, -77.9952)
  line L49 (-41.1289, -77.9952) -> (-31.1289, -77.9912)
  circle A64 centre (-117.2, -30) radius 2.425
  circle A65 centre (-117.2, -72) radius 2.425
  circle A66 centre (-183.2, -30) radius 2.425
  circle A67 centre (-183.2, -72) radius 2.425
  line L50 (-150.2, -24) -> (-183.9422, -24.0135)
  arc A68 (-187.8541, -22.1301) -> (-183.9422, -24.0135) centre (-183.9442, -19.0135) ccw
  arc A69 (-187.8541, -22.1301) -> (-192.0745, -26.3423) centre (-190.2, -24) ccw
  arc A70 (-190.1986, -30.2465) -> (-192.0745, -26.3423) centre (-195.1986, -30.2461) ccw
  line L51 (-190.1986, -30.2465) -> (-190.2, -51)
  line L52 (-190.2, -51) -> (-190.1996, -56.3768)
  line L53 (-190.1996, -56.3768) -> (-190.199, -66.3768)
  line L54 (-190.199, -66.3768) -> (-190.1986, -71.7535)
  arc A71 (-192.0745, -75.6577) -> (-190.1986, -71.7535) centre (-195.1986, -71.7539) ccw
  arc A72 (-192.0745, -75.6577) -> (-187.8541, -79.8699) centre (-190.2, -78) ccw
  arc A73 (-183.9422, -77.9865) -> (-187.8541, -79.8699) centre (-183.9442, -82.9865) ccw
  line L55 (-183.9422, -77.9865) -> (-172.0711, -77.9912)
  line L56 (-172.0711, -77.9912) -> (-162.0711, -77.9952)
  line L57 (-162.0711, -77.9952) -> (-150.2, -78)
  line L58 (-150.2, -78) -> (-116.4578, -77.9865)
  arc A74 (-112.5459, -79.8699) -> (-116.4578, -77.9865) centre (-116.4558, -82.9865) ccw
  arc A75 (-112.5459, -79.8699) -> (-108.3255, -75.6577) centre (-110.2, -78) ccw
  arc A76 (-110.2014, -71.7535) -> (-108.3255, -75.6577) centre (-105.2014, -71.7539) ccw
  line L59 (-110.2014, -71.7535) -> (-110.2, -51)
  line L60 (-110.2, -51) -> (-110.2014, -30.2465)
  arc A77 (-108.3255, -26.3423) -> (-110.2014, -30.2465) centre (-105.2014, -30.2461) ccw
  arc A78 (-108.3255, -26.3423) -> (-112.5459, -22.1301) centre (-110.2, -24) ccw
  arc A79 (-116.4578, -24.0135) -> (-112.5459, -22.1301) centre (-116.4558, -19.0135) ccw
  line L61 (-116.4578, -24.0135) -> (-150.2, -24)
  line L62 (-20, -33.425) -> (-20, -68.575) construction
  line L63 (-101.6, -203.2) -> (-101.6, 0) construction
  arc A80 (-20, -68.575) -> (-23.425, -72) centre (-20, -72) ccw construction
  line L64 (-23.425, -72) -> (-82.575, -72) construction
  arc A81 (-82.575, -72) -> (-86, -68.575) centre (-86, -72) ccw construction
  arc A82 (-86, -33.425) -> (-82.575, -30) centre (-86, -30) ccw construction
  line L65 (-86, -68.575) -> (-86, -33.425) construction
  arc A83 (-23.425, -30) -> (-20, -33.425) centre (-20, -30) ccw construction
  line L66 (-82.575, -30) -> (-23.425, -30) construction
  line L67 (-85, -67.6895) -> (-85, -34.3105)
  arc A84 (-85, -34.3105) -> (-81.6895, -31) centre (-86, -30) ccw
  line L68 (-81.6895, -31) -> (-24.3105, -31)
  arc A85 (-24.3105, -31) -> (-21, -34.3105) centre (-20, -30) ccw
  line L69 (-21, -34.3105) -> (-21, -67.6895)
  arc A86 (-21, -67.6895) -> (-24.3105, -71) centre (-20, -72) ccw
  line L70 (-24.3105, -71) -> (-81.6895, -71)
  arc A87 (-81.6895, -71) -> (-85, -67.6895) centre (-86, -72) ccw
  line L71 (-118.2, -67.6895) -> (-118.2, -34.3105)
  arc A88 (-121.5105, -31) -> (-118.2, -34.3105) centre (-117.2, -30) ccw
  line L72 (-121.5105, -31) -> (-178.8895, -31)
  arc A89 (-182.2, -34.3105) -> (-178.8895, -31) centre (-183.2, -30) ccw
  line L73 (-182.2, -34.3105) -> (-182.2, -67.6895)
  arc A90 (-178.8895, -71) -> (-182.2, -67.6895) centre (-183.2, -72) ccw
  line L74 (-178.8895, -71) -> (-121.5105, -71)
  arc A91 (-118.2, -67.6895) -> (-121.5105, -71) centre (-117.2, -72) ccw
  dimension "d78" = 1
  constraint horizontal L64
  constraint vertical L65
  constraint vertical L62
  constraint concentric A50 A80
  constraint concentric A48 A81
  constraint concentric A49 A82
  constraint concentric A51 A83
  constraint symmetric L63 L67.start L71.start
  constraint symmetric L63 L67.end L71.end
  constraint symmetric L63 A84.end A88.start
  constraint symmetric L63 A84 A88
  constraint symmetric L63 L68.end L72.end
  constraint symmetric L63 A85.end A89.start
  constraint symmetric L63 A85 A89
  constraint symmetric L63 L69.end L73.end
  constraint symmetric L63 A86.end A90.start
  constraint symmetric L63 A86 A90
  constraint symmetric L63 L70.end L74.end
  constraint symmetric L63 A87 A91
extrude "Extrude10" cut sketch "Sketch4" against normal blind 3 contours L67 A84 L68 A85 L69 A86 L70 A87 | L71 A88 L72 A89 L73 A90 L74 A91 bodies 1 in component "holder"
component "holder" placed x (1, 0, 0) y (0, 1, 0) z (0, 0, 1) at (0, 0, 0)
equation "d34 = ( 3.52 / 2 ) * 1 mm"
equation "d37 = d34"
equation "d43 = d39"
equation "d44 = d40"
equation "d64 = d60"
